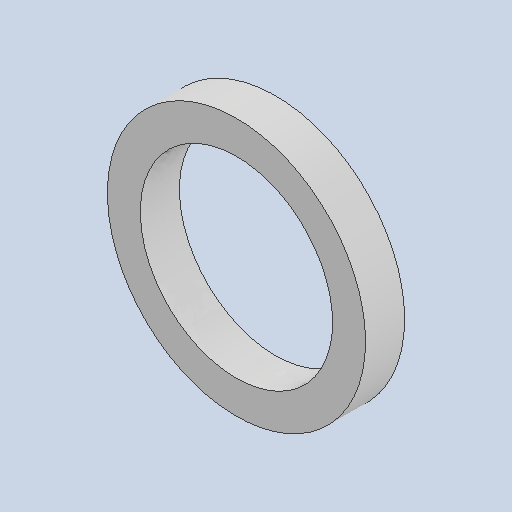
# Autodesk Inventor part: 177x35x10 bearing
Saved by Autodesk Inventor 2023 (Build 270158000, 158)
## iProperties
Created: 2023-01-17
Part Number: 177x35x10 bearing
Material: Generic
Document SubType Name: Modeling
Designer: caden
Density: 1 g/cm^3
Appearance: Default
Description: https://www.amazon.com/Othmro-6807-2RS-35x47x7mm-Accuracy-Bearing/dp/B081WW5JMM/ref=as_li_ss_tl?dchild=1&keywords=bearing%2B47x35&qid=1592496449&sr=8-4&linkCode=sl1&tag=ch-new-20&linkId=5da62ba0a0c68d1f5845c83534fe8526&language=en_US&th=1
Author: caden
Autodesk Inventor part; units mm, degrees
ref_plane "YZ Plane" through (0, 0, 0) normal (1, 0, 0) x (0, 1, 0)
ref_plane "XZ Plane" through (0, 0, 0) normal (0, 1, 0) x (-1, 0, 0)
ref_plane "XY Plane" through (0, 0, 0) normal (0, 0, 1) x (1, 0, 0)
sketch "Sketch1" plane through (0, 0, 0) normal (0, 0, 1) x (1, 0, 0)
  circle A0 centre (0, 0) radius 17.5
  circle A1 centre (0, 0) radius 23.495
  dimension "d0" = 35
  dimension "d1" = 46.99
  constraints: 2 centre point, 2 coincident
  measures "d0" diameter of A0
  measures "d1" diameter of A1
extrude "Extrusion1" add sketch "Sketch1" along normal blind 7.112
body "Solid1"
